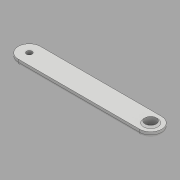
# Autodesk Inventor part: Link_2
Saved by Autodesk Inventor 2020 (Build 240168000, 168)
## iProperties
Created: 2020-02-20
Part Number: Link_2
Material: Generic
Document SubType Name: Modeling
Designer: Pece Jovanovski
Density: 1 g/cm^3
Appearance: Default
Mass: 0.0117854 g
Surface Area: 0.644248 cm^2
Volume: 0.0117854 cm^3
Author: Pece Jovanovski
Autodesk Inventor part; units mm, degrees
ref_plane "YZ Plane" through (0, 0, 0) normal (1, 0, 0) x (0, 1, 0)
ref_plane "XZ Plane" through (0, 0, 0) normal (0, 1, 0) x (-1, 0, 0)
ref_plane "XY Plane" through (0, 0, 0) normal (0, 0, 1) x (1, 0, 0)
sketch "Sketch1" plane through (0, 0, 0) normal (0, 0, 1) x (1, 0, 0)
  line L0 (-6.5, 1) -> (6.5, 1)
  line L1 (6.5, 1) -> (6.5, -1)
  line L2 (6.5, -1) -> (-6.5, -1)
  line L3 (-6.5, -1) -> (-6.5, 1)
  circle A0 centre (-5.5, 0) radius 0.25
  circle A1 centre (5.5, 0) radius 0.5
  point P0 (0, 0)
  point P1 (0, 1)
  point P2 (-6.5, 0)
  dimension "d0" = 2
  dimension "d1" = 0.5
  dimension "d2" = 1
  dimension "d7" = 13
  dimension "d8" = 1
  dimension "d12" = 1
  constraints: 8 end point, 3 horizontal alignment, 2 centre point, 2 midpoint, 2 parallel, 1 horizontal, 1 perpendicular, 1 vertical alignment
  measures "d0" distance between parallel lines of L2 L0
  measures "d1" diameter of A0
  measures "d2" diameter of A1
  measures "d7" distance of L0.start L0.end
  measures "d8" distance from line of A0.centre L3
  measures "d12" distance from line of L1 A1.centre
extrude "Extrusion1" add sketch "Sketch1" along normal mid plane 0.5
fillet "Fillet1" radius 1 4 edges at (6.5, 1, 0) (6.5, -1, 0) (-6.5, 1, 0) (-6.5, -1, 0)
sketch "Sketch3" plane through (0, 0, 0.25) normal (0, 0, 1) x (1, 0, 0)
  circle A0 centre (5.5, 0) radius 0.5 projected
  circle A1 centre (5.5, 0) radius 0.65
  point P0 (0, 0)
  dimension "d13" = 1.3
  constraints: 1 centre point, 1 coincident
  measures "d13" diameter of A1
extrude "Extrusion2" add sketch "Sketch3" along normal blind 0.15
chamfer "Chamfer1" distance 0.15 angle 45 1 edges at (4.85, 0, 0.4)
fillet "Fillet2" radius 0.25 8 edges at (-6.2071, 0.7071, -0.25) (-6.5, 0, -0.25) (-6.2071, -0.7071, -0.25) (0, 1, -0.25) (6.2071, 0.7071, -0.25) (6.5, 0, -0.25) (6.2071, -0.7071, -0.25) (0, -1, -0.25)
sketch "Sketch4" plane through (0, 0, -0.25) normal (0, 0, -1) x (-1, 0, 0)
  circle A0 centre (5.5, 0) radius 0.25 projected
  circle A1 centre (5.5, 0) radius 0.375
  point P0 (0, 0)
  dimension "d20" = 0.75
  constraints: 1 centre point, 1 coincident
  measures "d20" diameter of A1
extrude "Extrusion3" cut sketch "Sketch4" against normal blind 0.15
chamfer "Chamfer3" distance 0.1 angle 45 1 edges at (-5.125, 0, -0.25)
body "Solid1"
